Autodesk Fusion 360 part; units mm, degrees
(part 2 of 9)
sketch "草图7 (4)" plane through (0, 0, 36) normal (0, 0, 1) x (1, 0, 0) in component "L2_RemovableGrate"
  line L0 (299, 60.3) -> (303, 60.3)
  line L1 (303, 60.3) -> (303, 129.7)
  line L2 (303, 129.7) -> (299, 129.7)
  line L3 (299, 129.7) -> (299, 60.3)
  dimension "d526" = 299
  dimension "d528" = 4
  dimension "d529" = 69.4
  constraint horizontal L0
  constraint vertical L1
  constraint horizontal L2
  constraint vertical L3
  measures "d526" horizontal distance of origin L0.start
  measures "d528" horizontal distance of L0.start L0.end
  measures "d529" vertical distance of L0.end L1.end
extrude "Drain slot 6'" cut sketch "草图7 (4)" along normal blind 4 bodies 8 in component "L2_RemovableGrate"
ref_plane "工作平面8" through (0, 0, 36) normal (0, 0, 1) x (1, 0, 0) in component "L2_RemovableGrate"
sketch "草图8 (4)" plane through (0, 0, 36) normal (0, 0, 1) x (1, 0, 0) in component "L2_RemovableGrate"
  line L0 (309, 60.3) -> (313, 60.3)
  line L1 (313, 60.3) -> (313, 129.7)
  line L2 (313, 129.7) -> (309, 129.7)
  line L3 (309, 129.7) -> (309, 60.3)
  dimension "d534" = 309
  dimension "d536" = 4
  dimension "d537" = 69.4
  constraint horizontal L0
  constraint vertical L1
  constraint horizontal L2
  constraint vertical L3
  measures "d534" horizontal distance of origin L0.start
  measures "d536" horizontal distance of L0.start L0.end
  measures "d537" vertical distance of L0.end L1.end
extrude "Drain slot 7'" cut sketch "草图8 (4)" along normal blind 4 bodies 8 in component "L2_RemovableGrate"
ref_plane "工作平面9" through (0, 0, 36) normal (0, 0, 1) x (1, 0, 0) in component "L2_RemovableGrate"
sketch "草图9 (4)" plane through (0, 0, 36) normal (0, 0, 1) x (1, 0, 0) in component "L2_RemovableGrate"
  line L0 (319, 60.3) -> (323, 60.3)
  line L1 (323, 60.3) -> (323, 129.7)
  line L2 (323, 129.7) -> (319, 129.7)
  line L3 (319, 129.7) -> (319, 60.3)
  dimension "d542" = 319
  dimension "d544" = 4
  dimension "d545" = 69.4
  constraint horizontal L0
  constraint vertical L1
  constraint horizontal L2
  constraint vertical L3
  measures "d542" horizontal distance of origin L0.start
  measures "d544" horizontal distance of L0.start L0.end
  measures "d545" vertical distance of L0.end L1.end
extrude "Drain slot 8'" cut sketch "草图9 (4)" along normal blind 4 bodies 8 in component "L2_RemovableGrate"
ref_plane "工作平面10" through (0, 0, 36) normal (0, 0, 1) x (1, 0, 0) in component "L2_RemovableGrate"
sketch "草图10 (4)" plane through (0, 0, 36) normal (0, 0, 1) x (1, 0, 0) in component "L2_RemovableGrate"
  line L0 (329, 60.3) -> (333, 60.3)
  line L1 (333, 60.3) -> (333, 129.7)
  line L2 (333, 129.7) -> (329, 129.7)
  line L3 (329, 129.7) -> (329, 60.3)
  dimension "d550" = 329
  dimension "d552" = 4
  dimension "d553" = 69.4
  constraint horizontal L0
  constraint vertical L1
  constraint horizontal L2
  constraint vertical L3
  measures "d550" horizontal distance of origin L0.start
  measures "d552" horizontal distance of L0.start L0.end
  measures "d553" vertical distance of L0.end L1.end
extrude "Drain slot 9'" cut sketch "草图10 (4)" along normal blind 4 bodies 8 in component "L2_RemovableGrate"
ref_plane "工作平面11" through (0, 0, 36) normal (0, 0, 1) x (1, 0, 0) in component "L2_RemovableGrate"
sketch "草图11 (4)" plane through (0, 0, 36) normal (0, 0, 1) x (1, 0, 0) in component "L2_RemovableGrate"
  line L0 (339, 60.3) -> (343, 60.3)
  line L1 (343, 60.3) -> (343, 129.7)
  line L2 (343, 129.7) -> (339, 129.7)
  line L3 (339, 129.7) -> (339, 60.3)
  dimension "d558" = 339
  dimension "d560" = 4
  dimension "d561" = 69.4
  constraint horizontal L0
  constraint vertical L1
  constraint horizontal L2
  constraint vertical L3
  measures "d558" horizontal distance of origin L0.start
  measures "d560" horizontal distance of L0.start L0.end
  measures "d561" vertical distance of L0.end L1.end
extrude "Drain slot 10'" cut sketch "草图11 (4)" along normal blind 4 bodies 8 in component "L2_RemovableGrate"
ref_plane "工作平面12" through (0, 0, 36) normal (0, 0, 1) x (1, 0, 0) in component "L2_RemovableGrate"
sketch "草图12 (4)" plane through (0, 0, 36) normal (0, 0, 1) x (1, 0, 0) in component "L2_RemovableGrate"
  line L0 (349, 60.3) -> (353, 60.3)
  line L1 (353, 60.3) -> (353, 129.7)
  line L2 (353, 129.7) -> (349, 129.7)
  line L3 (349, 129.7) -> (349, 60.3)
  dimension "d566" = 349
  dimension "d568" = 4
  dimension "d569" = 69.4
  constraint horizontal L0
  constraint vertical L1
  constraint horizontal L2
  constraint vertical L3
  measures "d566" horizontal distance of origin L0.start
  measures "d568" horizontal distance of L0.start L0.end
  measures "d569" vertical distance of L0.end L1.end
extrude "Drain slot 11'" cut sketch "草图12 (4)" along normal blind 4 bodies 8 in component "L2_RemovableGrate"
ref_plane "工作平面13" through (0, 0, 36) normal (0, 0, 1) x (1, 0, 0) in component "L2_RemovableGrate"
sketch "草图13 (4)" plane through (0, 0, 36) normal (0, 0, 1) x (1, 0, 0) in component "L2_RemovableGrate"
  line L0 (359, 60.3) -> (363, 60.3)
  line L1 (363, 60.3) -> (363, 129.7)
  line L2 (363, 129.7) -> (359, 129.7)
  line L3 (359, 129.7) -> (359, 60.3)
  dimension "d574" = 359
  dimension "d576" = 4
  dimension "d577" = 69.4
  constraint horizontal L0
  constraint vertical L1
  constraint horizontal L2
  constraint vertical L3
  measures "d574" horizontal distance of origin L0.start
  measures "d576" horizontal distance of L0.start L0.end
  measures "d577" vertical distance of L0.end L1.end
extrude "Drain slot 12'" cut sketch "草图13 (4)" along normal blind 4 bodies 8 in component "L2_RemovableGrate"
ref_plane "工作平面14" through (0, 0, 36) normal (0, 0, 1) x (1, 0, 0) in component "L2_RemovableGrate"
sketch "草图14 (4)" plane through (0, 0, 36) normal (0, 0, 1) x (1, 0, 0) in component "L2_RemovableGrate"
  line L0 (369, 60.3) -> (373, 60.3)
  line L1 (373, 60.3) -> (373, 129.7)
  line L2 (373, 129.7) -> (369, 129.7)
  line L3 (369, 129.7) -> (369, 60.3)
  dimension "d582" = 369
  dimension "d584" = 4
  dimension "d585" = 69.4
  constraint horizontal L0
  constraint vertical L1
  constraint horizontal L2
  constraint vertical L3
  measures "d582" horizontal distance of origin L0.start
  measures "d584" horizontal distance of L0.start L0.end
  measures "d585" vertical distance of L0.end L1.end
extrude "Drain slot 13'" cut sketch "草图14 (4)" along normal blind 4 bodies 8 in component "L2_RemovableGrate"
ref_plane "工作平面15" through (0, 0, 36) normal (0, 0, 1) x (1, 0, 0) in component "L2_RemovableGrate"
sketch "草图15 (4)" plane through (0, 0, 36) normal (0, 0, 1) x (1, 0, 0) in component "L2_RemovableGrate"
  line L0 (379, 60.3) -> (383, 60.3)
  line L1 (383, 60.3) -> (383, 129.7)
  line L2 (383, 129.7) -> (379, 129.7)
  line L3 (379, 129.7) -> (379, 60.3)
  dimension "d590" = 379
  dimension "d592" = 4
  dimension "d593" = 69.4
  constraint horizontal L0
  constraint vertical L1
  constraint horizontal L2
  constraint vertical L3
  measures "d590" horizontal distance of origin L0.start
  measures "d592" horizontal distance of L0.start L0.end
  measures "d593" vertical distance of L0.end L1.end
extrude "Drain slot 14" cut sketch "草图15 (4)" along normal blind 4 bodies 8 in component "L2_RemovableGrate"
ref_plane "工作平面16" through (0, 0, 36) normal (0, 0, 1) x (1, 0, 0) in component "L2_RemovableGrate"
sketch "草图16" plane through (0, 0, 36) normal (0, 0, 1) x (1, 0, 0) in component "L2_RemovableGrate"
  line L0 (389, 60.3) -> (393, 60.3)
  line L1 (393, 60.3) -> (393, 129.7)
  line L2 (393, 129.7) -> (389, 129.7)
  line L3 (389, 129.7) -> (389, 60.3)
  dimension "d598" = 389
  dimension "d600" = 4
  dimension "d601" = 69.4
  constraint horizontal L0
  constraint vertical L1
  constraint horizontal L2
  constraint vertical L3
  measures "d598" horizontal distance of origin L0.start
  measures "d600" horizontal distance of L0.start L0.end
  measures "d601" vertical distance of L0.end L1.end
extrude "Drain slot 15" cut sketch "草图16" along normal blind 4 bodies 8 in component "L2_RemovableGrate"
ref_plane "工作平面17" through (0, 0, 36) normal (0, 0, 1) x (1, 0, 0) in component "L2_RemovableGrate"
sketch "草图17" plane through (0, 0, 36) normal (0, 0, 1) x (1, 0, 0) in component "L2_RemovableGrate"
  line L0 (399, 60.3) -> (403, 60.3)
  line L1 (403, 60.3) -> (403, 129.7)
  line L2 (403, 129.7) -> (399, 129.7)
  line L3 (399, 129.7) -> (399, 60.3)
  dimension "d606" = 399
  dimension "d608" = 4
  dimension "d609" = 69.4
  constraint horizontal L0
  constraint vertical L1
  constraint horizontal L2
  constraint vertical L3
  measures "d606" horizontal distance of origin L0.start
  measures "d608" horizontal distance of L0.start L0.end
  measures "d609" vertical distance of L0.end L1.end
extrude "Drain slot 16" cut sketch "草图17" along normal blind 4 bodies 8 in component "L2_RemovableGrate"
ref_plane "工作平面18" through (0, 0, 36) normal (0, 0, 1) x (1, 0, 0) in component "L2_RemovableGrate"
sketch "草图18" plane through (0, 0, 36) normal (0, 0, 1) x (1, 0, 0) in component "L2_RemovableGrate"
  line L0 (409, 60.3) -> (413, 60.3)
  line L1 (413, 60.3) -> (413, 129.7)
  line L2 (413, 129.7) -> (409, 129.7)
  line L3 (409, 129.7) -> (409, 60.3)
  dimension "d614" = 409
  dimension "d616" = 4
  dimension "d617" = 69.4
  constraint horizontal L0
  constraint vertical L1
  constraint horizontal L2
  constraint vertical L3
  measures "d614" horizontal distance of origin L0.start
  measures "d616" horizontal distance of L0.start L0.end
  measures "d617" vertical distance of L0.end L1.end
extrude "Drain slot 17" cut sketch "草图18" along normal blind 4 bodies 8 in component "L2_RemovableGrate"
ref_plane "工作平面19" through (0, 0, 36) normal (0, 0, 1) x (1, 0, 0) in component "L2_RemovableGrate"
sketch "草图19" plane through (0, 0, 36) normal (0, 0, 1) x (1, 0, 0) in component "L2_RemovableGrate"
  line L0 (323, 132.7) -> (339, 132.7)
  line L1 (339, 132.7) -> (339, 137.7)
  line L2 (339, 137.7) -> (323, 137.7)
  line L3 (323, 137.7) -> (323, 132.7)
  dimension "d622" = 323
  dimension "d623" = 132.7
  dimension "d624" = 16
  dimension "d625" = 5
  constraint horizontal L0
  constraint vertical L1
  constraint horizontal L2
  constraint vertical L3
  measures "d622" horizontal distance of origin L0.start
  measures "d623" vertical distance of origin L0.start
  measures "d624" horizontal distance of L0.start L0.end
  measures "d625" vertical distance of L0.end L1.end
extrude "Finger lift notch'" cut sketch "草图19" along normal blind 4 bodies 8 in component "L2_RemovableGrate"
ref_plane "工作平面1" through (0, 0, 0) normal (0, 0, 1) x (1, 0, 0) in component "L2_Foot_00"
sketch "草图1 (9)" plane through (0, 0, 0) normal (0, 0, 1) x (1, 0, 0) in component "L2_Foot_00"
  line L0 (235, 53) -> (251, 53)
  line L1 (251, 53) -> (251, 69)
  line L2 (251, 69) -> (235, 69)
  line L3 (235, 69) -> (235, 53)
  dimension "d630" = 235
  dimension "d631" = 53
  dimension "d632" = 16
  dimension "d633" = 16
  constraint horizontal L0
  constraint vertical L1
  constraint horizontal L2
  constraint vertical L3
  measures "d630" horizontal distance of origin L0.start
  measures "d631" vertical distance of origin L0.start
  measures "d632" horizontal distance of L0.start L0.end
  measures "d633" vertical distance of L0.end L1.end
extrude "Foot base''''" add sketch "草图1 (9)" along normal blind 20 separate body makes body 9 in component "L2_Foot_00"
ref_plane "工作平面2" through (0, 0, 20) normal (0, 0, 1) x (1, 0, 0) in component "L2_Foot_00"
sketch "草图2 (9)" plane through (0, 0, 20) normal (0, 0, 1) x (1, 0, 0) in component "L2_Foot_00"
  line L0 (239, 57) -> (247, 57)
  line L1 (247, 57) -> (247, 65)
  line L2 (247, 65) -> (239, 65)
  line L3 (239, 65) -> (239, 57)
  dimension "d638" = 239
  dimension "d639" = 57
  dimension "d640" = 8
  dimension "d641" = 8
  constraint horizontal L0
  constraint vertical L1
  constraint horizontal L2
  constraint vertical L3
  measures "d638" horizontal distance of origin L0.start
  measures "d639" vertical distance of origin L0.start
  measures "d640" horizontal distance of L0.start L0.end
  measures "d641" vertical distance of L0.end L1.end
extrude "Locating peg''''" add sketch "草图2 (9)" along normal blind 1.5 bodies 9 in component "L2_Foot_00"
ref_plane "工作平面1" through (0, 0, 0) normal (0, 0, 1) x (1, 0, 0) in component "L2_Foot_01"
sketch "草图1 (10)" plane through (0, 0, 0) normal (0, 0, 1) x (1, 0, 0) in component "L2_Foot_01"
  line L0 (235, 115) -> (251, 115)
  line L1 (251, 115) -> (251, 131)
  line L2 (251, 131) -> (235, 131)
  line L3 (235, 131) -> (235, 115)
  dimension "d646" = 235
  dimension "d647" = 115
  dimension "d648" = 16
  dimension "d649" = 16
  constraint horizontal L0
  constraint vertical L1
  constraint horizontal L2
  constraint vertical L3
  measures "d646" horizontal distance of origin L0.start
  measures "d647" vertical distance of origin L0.start
  measures "d648" horizontal distance of L0.start L0.end
  measures "d649" vertical distance of L0.end L1.end
extrude "Foot base'''''" add sketch "草图1 (10)" along normal blind 20 separate body makes body 10 in component "L2_Foot_01"
ref_plane "工作平面2" through (0, 0, 20) normal (0, 0, 1) x (1, 0, 0) in component "L2_Foot_01"
sketch "草图2 (10)" plane through (0, 0, 20) normal (0, 0, 1) x (1, 0, 0) in component "L2_Foot_01"
  line L0 (239, 119) -> (247, 119)
  line L1 (247, 119) -> (247, 127)
  line L2 (247, 127) -> (239, 127)
  line L3 (239, 127) -> (239, 119)
  dimension "d654" = 239
  dimension "d655" = 119
  dimension "d656" = 8
  dimension "d657" = 8
  constraint horizontal L0
  constraint vertical L1
  constraint horizontal L2
  constraint vertical L3
  measures "d654" horizontal distance of origin L0.start
  measures "d655" vertical distance of origin L0.start
  measures "d656" horizontal distance of L0.start L0.end
  measures "d657" vertical distance of L0.end L1.end
extrude "Locating peg'''''" add sketch "草图2 (10)" along normal blind 1.5 bodies 10 in component "L2_Foot_01"
ref_plane "工作平面1" through (0, 0, 0) normal (0, 0, 1) x (1, 0, 0) in component "L2_Foot_10"
sketch "草图1 (11)" plane through (0, 0, 0) normal (0, 0, 1) x (1, 0, 0) in component "L2_Foot_10"
  line L0 (411, 53) -> (427, 53)
  line L1 (427, 53) -> (427, 69)
  line L2 (427, 69) -> (411, 69)
  line L3 (411, 69) -> (411, 53)
  dimension "d662" = 411
  dimension "d663" = 53
  dimension "d664" = 16
  dimension "d665" = 16
  constraint horizontal L0
  constraint vertical L1
  constraint horizontal L2
  constraint vertical L3
  measures "d662" horizontal distance of origin L0.start
  measures "d663" vertical distance of origin L0.start
  measures "d664" horizontal distance of L0.start L0.end
  measures "d665" vertical distance of L0.end L1.end
extrude "Foot base''''''" add sketch "草图1 (11)" along normal blind 20 separate body makes body 11 in component "L2_Foot_10"
ref_plane "工作平面2" through (0, 0, 20) normal (0, 0, 1) x (1, 0, 0) in component "L2_Foot_10"
sketch "草图2 (11)" plane through (0, 0, 20) normal (0, 0, 1) x (1, 0, 0) in component "L2_Foot_10"
  line L0 (415, 57) -> (423, 57)
  line L1 (423, 57) -> (423, 65)
  line L2 (423, 65) -> (415, 65)
  line L3 (415, 65) -> (415, 57)
  dimension "d670" = 415
  dimension "d671" = 57
  dimension "d672" = 8
  dimension "d673" = 8
  constraint horizontal L0
  constraint vertical L1
  constraint horizontal L2
  constraint vertical L3
  measures "d670" horizontal distance of origin L0.start
  measures "d671" vertical distance of origin L0.start
  measures "d672" horizontal distance of L0.start L0.end
  measures "d673" vertical distance of L0.end L1.end
extrude "Locating peg''''''" add sketch "草图2 (11)" along normal blind 1.5 bodies 11 in component "L2_Foot_10"
ref_plane "工作平面1" through (0, 0, 0) normal (0, 0, 1) x (1, 0, 0) in component "L2_Foot_11"
sketch "草图1 (12)" plane through (0, 0, 0) normal (0, 0, 1) x (1, 0, 0) in component "L2_Foot_11"
  line L0 (411, 115) -> (427, 115)
  line L1 (427, 115) -> (427, 131)
  line L2 (427, 131) -> (411, 131)
  line L3 (411, 131) -> (411, 115)
  dimension "d678" = 411
  dimension "d679" = 115
  dimension "d680" = 16
  dimension "d681" = 16
  constraint horizontal L0
  constraint vertical L1
  constraint horizontal L2
  constraint vertical L3
  measures "d678" horizontal distance of origin L0.start
  measures "d679" vertical distance of origin L0.start
  measures "d680" horizontal distance of L0.start L0.end
  measures "d681" vertical distance of L0.end L1.end
extrude "Foot base'''''''" add sketch "草图1 (12)" along normal blind 20 separate body makes body 12 in component "L2_Foot_11"
ref_plane "工作平面2" through (0, 0, 20) normal (0, 0, 1) x (1, 0, 0) in component "L2_Foot_11"
sketch "草图2 (12)" plane through (0, 0, 20) normal (0, 0, 1) x (1, 0, 0) in component "L2_Foot_11"
  line L0 (415, 119) -> (423, 119)
  line L1 (423, 119) -> (423, 127)
  line L2 (423, 127) -> (415, 127)
  line L3 (415, 127) -> (415, 119)
  dimension "d686" = 415
  dimension "d687" = 119
  dimension "d688" = 8
  dimension "d689" = 8
  constraint horizontal L0
  constraint vertical L1
  constraint horizontal L2
  constraint vertical L3
  measures "d686" horizontal distance of origin L0.start
  measures "d687" vertical distance of origin L0.start
  measures "d688" horizontal distance of L0.start L0.end
  measures "d689" vertical distance of L0.end L1.end
extrude "Locating peg'''''''" add sketch "草图2 (12)" along normal blind 1.5 bodies 12 in component "L2_Foot_11"
ref_plane "工作平面1" through (0, 0, 20) normal (0, 0, 1) x (1, 0, 0) in component "R1_DrainPan"
sketch "草图1 (13)" plane through (0, 0, 20) normal (0, 0, 1) x (1, 0, 0) in component "R1_DrainPan"
  line L0 (590, 50) -> (724, 50)
  line L1 (724, 50) -> (724, 140)
  line L2 (724, 140) -> (590, 140)
  line L3 (590, 140) -> (590, 50)
  dimension "d694" = 590
  dimension "d695" = 50
  dimension "d696" = 134
  dimension "d697" = 90
  constraint horizontal L0
  constraint vertical L1
  constraint horizontal L2
  constraint vertical L3
  measures "d694" horizontal distance of origin L0.start
  measures "d695" vertical distance of origin L0.start
  measures "d696" horizontal distance of L0.start L0.end
  measures "d697" vertical distance of L0.end L1.end
extrude "Pan blank''" add sketch "草图1 (13)" along normal blind 20 separate body makes body 13 in component "R1_DrainPan"
fillet "Outside corner rounds''" radius 3 4 edges at (590, 140, 30) (724, 140, 30) (724, 50, 30) (590, 50, 30) on bodies 13 in component "R1_DrainPan"
ref_plane "工作平面2" through (593, 0, 0) normal (1, 0, 0) x (0, 1, 0) in component "R1_DrainPan"
sketch "草图2 (13)" plane through (593, 0, 0) normal (1, 0, 0) x (0, 0, -1) in component "R1_DrainPan"
  line L0 (-30.8318, 53) -> (-24.958, 137)
  line L1 (-24.958, 137) -> (-41, 137)
  line L2 (-41, 137) -> (-41, 53)
  line L3 (-41, 53) -> (-30.8318, 53)
  dimension "d704" = 30.8318
  dimension "d706" = 24.958
  dimension "d708" = 41
  constraint horizontal L1
  constraint vertical L2
  constraint horizontal L3
  measures "d704" horizontal distance of origin L0.start
  measures "d706" horizontal distance of origin L0.end
  measures "d708" horizontal distance of origin L1.end
extrude "Sloped catch cavity''" cut sketch "草图2 (13)" along normal blind 128 bodies 13 in component "R1_DrainPan"
ref_plane "工作平面3" through (640, 0, 0) normal (1, 0, 0) x (0, 1, 0) in component "R1_DrainPan"
sketch "草图3 (5)" plane through (640, 0, 0) normal (1, 0, 0) x (0, 0, -1) in component "R1_DrainPan"
  line L0 (-20, 137) -> (-20, 165)
  line L1 (-20, 165) -> (-23, 165)
  line L2 (-23, 165) -> (-24.958, 137)
  line L3 (-24.958, 137) -> (-20, 137)
  dimension "d716" = 23
  dimension "d717" = 24.958
  constraint vertical L0
  constraint horizontal L1
  constraint horizontal L3
  measures "d716" horizontal distance of origin L1.end
  measures "d717" horizontal distance of origin L2.end
extrude "Drain tongue floor''" add sketch "草图3 (5)" along normal blind 34 bodies 13 in component "R1_DrainPan"
ref_plane "工作平面4" through (640, 0, 0) normal (1, 0, 0) x (0, 1, 0) in component "R1_DrainPan"
sketch "草图4 (5)" plane through (640, 0, 0) normal (1, 0, 0) x (0, 0, -1) in component "R1_DrainPan"
  line L0 (-20, 137) -> (-20, 165)
  line L1 (-20, 165) -> (-29, 165)
  line L2 (-29, 165) -> (-30.958, 137)
  line L3 (-30.958, 137) -> (-20, 137)
  dimension "d725" = 29
  dimension "d726" = 30.958
  constraint vertical L0
  constraint horizontal L1
  constraint horizontal L3
  measures "d725" horizontal distance of origin L1.end
  measures "d726" horizontal distance of origin L2.end
extrude "Tongue side rail''" add sketch "草图4 (5)" along normal blind 3 bodies 13 in component "R1_DrainPan"
ref_plane "工作平面5" through (671, 0, 0) normal (1, 0, 0) x (0, 1, 0) in component "R1_DrainPan"
sketch "草图5 (5)" plane through (671, 0, 0) normal (1, 0, 0) x (0, 0, -1) in component "R1_DrainPan"
  line L0 (-20, 137) -> (-20, 165)
  line L1 (-20, 165) -> (-29, 165)
  line L2 (-29, 165) -> (-30.958, 137)
  line L3 (-30.958, 137) -> (-20, 137)
  dimension "d734" = 29
  dimension "d735" = 30.958
  constraint vertical L0
  constraint horizontal L1
  constraint horizontal L3
  measures "d734" horizontal distance of origin L1.end
  measures "d735" horizontal distance of origin L2.end
extrude "Tongue side rail (1)''" add sketch "草图5 (5)" along normal blind 3 bodies 13 in component "R1_DrainPan"
ref_plane "工作平面6" through (643, 0, 0) normal (1, 0, 0) x (0, 1, 0) in component "R1_DrainPan"
sketch "草图6 (5)" plane through (643, 0, 0) normal (1, 0, 0) x (0, 0, -1) in component "R1_DrainPan"
  line L0 (-24.958, 137) -> (-23, 165)
  line L1 (-23, 165) -> (-41, 165)
  line L2 (-41, 165) -> (-41, 137)
  line L3 (-41, 137) -> (-24.958, 137)
  dimension "d740" = 24.958
  dimension "d742" = 23
  dimension "d744" = 41
  constraint horizontal L1
  constraint vertical L2
  constraint horizontal L3
  measures "d740" horizontal distance of origin L0.start
  measures "d742" horizontal distance of origin L0.end
  measures "d744" horizontal distance of origin L1.end
extrude "Open drain mouth''" cut sketch "草图6 (5)" along normal blind 28 bodies 13 in component "R1_DrainPan"
ref_plane "工作平面7" through (0, 0, 20) normal (0, 0, 1) x (1, 0, 0) in component "R1_DrainPan"
sketch "草图7 (5)" plane through (0, 0, 20) normal (0, 0, 1) x (1, 0, 0) in component "R1_DrainPan"
  line L0 (593, 53) -> (605, 53)
  line L1 (605, 53) -> (605, 65)
  line L2 (605, 65) -> (593, 65)
  line L3 (593, 65) -> (593, 53)
  dimension "d751" = 12
  dimension "d752" = 12
  constraint horizontal L0
  constraint vertical L1
  constraint horizontal L2
  constraint vertical L3
  measures "d751" horizontal distance of L0.start L0.end
  measures "d752" vertical distance of L0.end L1.end
extrude "Grate seat 00''" add sketch "草图7 (5)" along normal blind 16 bodies 13 in component "R1_DrainPan"
ref_plane "工作平面8" through (0, 0, 20) normal (0, 0, 1) x (1, 0, 0) in component "R1_DrainPan"
sketch "草图8 (5)" plane through (0, 0, 20) normal (0, 0, 1) x (1, 0, 0) in component "R1_DrainPan"
  line L0 (593, 125) -> (605, 125)
  line L1 (605, 125) -> (605, 137)
  line L2 (605, 137) -> (593, 137)
  line L3 (593, 137) -> (593, 125)
  dimension "d758" = 125
  dimension "d759" = 12
  dimension "d760" = 12
  constraint horizontal L0
  constraint vertical L1
  constraint horizontal L2
  constraint vertical L3
  measures "d758" vertical distance of origin L0.start
  measures "d759" horizontal distance of L0.start L0.end
  measures "d760" vertical distance of L0.end L1.end
extrude "Grate seat 01''" add sketch "草图8 (5)" along normal blind 16 bodies 13 in component "R1_DrainPan"
ref_plane "工作平面9" through (0, 0, 20) normal (0, 0, 1) x (1, 0, 0) in component "R1_DrainPan"
sketch "草图9 (5)" plane through (0, 0, 20) normal (0, 0, 1) x (1, 0, 0) in component "R1_DrainPan"
  line L0 (709, 53) -> (721, 53)
  line L1 (721, 53) -> (721, 65)
  line L2 (721, 65) -> (709, 65)
  line L3 (709, 65) -> (709, 53)
  dimension "d765" = 709
  dimension "d767" = 12
  dimension "d768" = 12
  constraint horizontal L0
  constraint vertical L1
  constraint horizontal L2
  constraint vertical L3
  measures "d765" horizontal distance of origin L0.start
  measures "d767" horizontal distance of L0.start L0.end
  measures "d768" vertical distance of L0.end L1.end
extrude "Grate seat 10''" add sketch "草图9 (5)" along normal blind 16 bodies 13 in component "R1_DrainPan"
ref_plane "工作平面10" through (0, 0, 20) normal (0, 0, 1) x (1, 0, 0) in component "R1_DrainPan"
sketch "草图10 (5)" plane through (0, 0, 20) normal (0, 0, 1) x (1, 0, 0) in component "R1_DrainPan"
  line L0 (709, 125) -> (721, 125)
  line L1 (721, 125) -> (721, 137)
  line L2 (721, 137) -> (709, 137)
  line L3 (709, 137) -> (709, 125)
  dimension "d773" = 709
  dimension "d774" = 125
  dimension "d775" = 12
  dimension "d776" = 12
  constraint horizontal L0
  constraint vertical L1
  constraint horizontal L2
  constraint vertical L3
  measures "d773" horizontal distance of origin L0.start
  measures "d774" vertical distance of origin L0.start
  measures "d775" horizontal distance of L0.start L0.end
  measures "d776" vertical distance of L0.end L1.end
extrude "Grate seat 11''" add sketch "草图10 (5)" along normal blind 16 bodies 13 in component "R1_DrainPan"
ref_plane "工作平面11" through (640, 0, 0) normal (1, 0, 0) x (0, 1, 0) in component "R1_DrainPan"
sketch "草图11 (5)" plane through (640, 0, 0) normal (1, 0, 0) x (0, 0, -1) in component "R1_DrainPan"
  line L0 (-19.8, 163) -> (-19.8, 164)
  line L1 (-19.8, 164) -> (-20.6, 164)
  line L2 (-20.6, 164) -> (-20.6, 163)
  line L3 (-20.6, 163) -> (-19.8, 163)
  dimension "d781" = 19.8
  dimension "d782" = 163
  dimension "d783" = 164
  dimension "d784" = 20.6
  constraint vertical L0
  constraint horizontal L1
  constraint vertical L2
  constraint horizontal L3
  measures "d781" horizontal distance of origin L0.start
  measures "d782" vertical distance of origin L0.start
  measures "d783" vertical distance of origin L0.end
  measures "d784" horizontal distance of origin L1.end
extrude "Drip break underside groove''" cut sketch "草图11 (5)" along normal blind 34 bodies 13 in component "R1_DrainPan"
ref_plane "工作平面12" through (0, 0, 20) normal (0, 0, 1) x (1, 0, 0) in component "R1_DrainPan"
sketch "草图12 (5)" plane through (0, 0, 20) normal (0, 0, 1) x (1, 0, 0) in component "R1_DrainPan"
  line L0 (596.75, 56.75) -> (605.25, 56.75)
  line L1 (605.25, 56.75) -> (605.25, 65.25)
  line L2 (605.25, 65.25) -> (596.75, 65.25)
  line L3 (596.75, 65.25) -> (596.75, 56.75)
  dimension "d789" = 596.75
  dimension "d790" = 56.75
  dimension "d791" = 8.5
  dimension "d792" = 8.5
  constraint horizontal L0
  constraint vertical L1
  constraint horizontal L2
  constraint vertical L3
  measures "d789" horizontal distance of origin L0.start
  measures "d790" vertical distance of origin L0.start
  measures "d791" horizontal distance of L0.start L0.end
  measures "d792" vertical distance of L0.end L1.end
extrude "Foot socket 00''" cut sketch "草图12 (5)" along normal blind 1.8 bodies 13 in component "R1_DrainPan"
ref_plane "工作平面13" through (0, 0, 20) normal (0, 0, 1) x (1, 0, 0) in component "R1_DrainPan"
sketch "草图13 (5)" plane through (0, 0, 20) normal (0, 0, 1) x (1, 0, 0) in component "R1_DrainPan"
  line L0 (596.75, 118.75) -> (605.25, 118.75)
  line L1 (605.25, 118.75) -> (605.25, 127.25)
  line L2 (605.25, 127.25) -> (596.75, 127.25)
  line L3 (596.75, 127.25) -> (596.75, 118.75)
  dimension "d797" = 596.75
  dimension "d798" = 118.75
  dimension "d799" = 8.5
  dimension "d800" = 8.5
  constraint horizontal L0
  constraint vertical L1
  constraint horizontal L2
  constraint vertical L3
  measures "d797" horizontal distance of origin L0.start
  measures "d798" vertical distance of origin L0.start
  measures "d799" horizontal distance of L0.start L0.end
  measures "d800" vertical distance of L0.end L1.end
extrude "Foot socket 01''" cut sketch "草图13 (5)" along normal blind 1.8 bodies 13 in component "R1_DrainPan"
ref_plane "工作平面14" through (0, 0, 20) normal (0, 0, 1) x (1, 0, 0) in component "R1_DrainPan"
sketch "草图14 (5)" plane through (0, 0, 20) normal (0, 0, 1) x (1, 0, 0) in component "R1_DrainPan"
  line L0 (708.75, 56.75) -> (717.25, 56.75)
  line L1 (717.25, 56.75) -> (717.25, 65.25)
  line L2 (717.25, 65.25) -> (708.75, 65.25)
  line L3 (708.75, 65.25) -> (708.75, 56.75)
  dimension "d805" = 708.75
  dimension "d806" = 56.75
  dimension "d807" = 8.5
  dimension "d808" = 8.5
  constraint horizontal L0
  constraint vertical L1
  constraint horizontal L2
  constraint vertical L3
  measures "d805" horizontal distance of origin L0.start
  measures "d806" vertical distance of origin L0.start
  measures "d807" horizontal distance of L0.start L0.end
  measures "d808" vertical distance of L0.end L1.end
extrude "Foot socket 10''" cut sketch "草图14 (5)" along normal blind 1.8 bodies 13 in component "R1_DrainPan"
ref_plane "工作平面15" through (0, 0, 20) normal (0, 0, 1) x (1, 0, 0) in component "R1_DrainPan"
sketch "草图15 (5)" plane through (0, 0, 20) normal (0, 0, 1) x (1, 0, 0) in component "R1_DrainPan"
  line L0 (708.75, 118.75) -> (717.25, 118.75)
  line L1 (717.25, 118.75) -> (717.25, 127.25)
  line L2 (717.25, 127.25) -> (708.75, 127.25)
  line L3 (708.75, 127.25) -> (708.75, 118.75)
  dimension "d813" = 708.75
  dimension "d814" = 118.75
  dimension "d815" = 8.5
  dimension "d816" = 8.5
  constraint horizontal L0
  constraint vertical L1
  constraint horizontal L2
  constraint vertical L3
  measures "d813" horizontal distance of origin L0.start
  measures "d814" vertical distance of origin L0.start
  measures "d815" horizontal distance of L0.start L0.end
  measures "d764" distance of L0.end L1.end
extrude "Foot socket 11''" cut sketch "草图15 (5)" along normal blind 1.8 bodies 13 in component "R1_DrainPan"
ref_plane "工作平面1" through (0, 0, 36) normal (0, 0, 1) x (1, 0, 0) in component "R1_RemovableGrate"
sketch "草图1 (14)" plane through (0, 0, 36) normal (0, 0, 1) x (1, 0, 0) in component "R1_RemovableGrate"
  line L0 (593.3, 53.3) -> (720.7, 53.3)
  line L1 (720.7, 53.3) -> (720.7, 136.7)
  line L2 (720.7, 136.7) -> (593.3, 136.7)
  line L3 (593.3, 136.7) -> (593.3, 53.3)
  dimension "d823" = 127.4
  dimension "d824" = 83.4
  constraint horizontal L0
  constraint vertical L1
  constraint horizontal L2
  constraint vertical L3
  measures "d823" horizontal distance of L0.start L0.end
  measures "d824" vertical distance of L0.end L1.end
extrude "Horizontal removable deck''" add sketch "草图1 (14)" along normal blind 4 separate body makes body 14 in component "R1_RemovableGrate"
ref_plane "工作平面2" through (0, 0, 36) normal (0, 0, 1) x (1, 0, 0) in component "R1_RemovableGrate"
sketch "草图2 (14)" plane through (0, 0, 36) normal (0, 0, 1) x (1, 0, 0) in component "R1_RemovableGrate"
  line L0 (605, 60.3) -> (609, 60.3)
  line L1 (609, 60.3) -> (609, 129.7)
  line L2 (609, 129.7) -> (605, 129.7)
  line L3 (605, 129.7) -> (605, 60.3)
  dimension "d829" = 605
  dimension "d831" = 4
  dimension "d832" = 69.4
  constraint horizontal L0
  constraint vertical L1
  constraint horizontal L2
  constraint vertical L3
  measures "d829" horizontal distance of origin L0.start
  measures "d831" horizontal distance of L0.start L0.end
  measures "d832" vertical distance of L0.end L1.end
extrude "Drain slot 1''" cut sketch "草图2 (14)" along normal blind 4 bodies 14 in component "R1_RemovableGrate"
ref_plane "工作平面3" through (0, 0, 36) normal (0, 0, 1) x (1, 0, 0) in component "R1_RemovableGrate"
sketch "草图3 (6)" plane through (0, 0, 36) normal (0, 0, 1) x (1, 0, 0) in component "R1_RemovableGrate"
  line L0 (615, 60.3) -> (619, 60.3)
  line L1 (619, 60.3) -> (619, 129.7)
  line L2 (619, 129.7) -> (615, 129.7)
  line L3 (615, 129.7) -> (615, 60.3)
  dimension "d837" = 615
  dimension "d839" = 4
  dimension "d840" = 69.4
  constraint horizontal L0
  constraint vertical L1
  constraint horizontal L2
  constraint vertical L3
  measures "d837" horizontal distance of origin L0.start
  measures "d839" horizontal distance of L0.start L0.end
  measures "d840" vertical distance of L0.end L1.end
extrude "Drain slot 2''" cut sketch "草图3 (6)" along normal blind 4 bodies 14 in component "R1_RemovableGrate"
ref_plane "工作平面4" through (0, 0, 36) normal (0, 0, 1) x (1, 0, 0) in component "R1_RemovableGrate"
sketch "草图4 (6)" plane through (0, 0, 36) normal (0, 0, 1) x (1, 0, 0) in component "R1_RemovableGrate"
  line L0 (625, 60.3) -> (629, 60.3)
  line L1 (629, 60.3) -> (629, 129.7)
  line L2 (629, 129.7) -> (625, 129.7)
  line L3 (625, 129.7) -> (625, 60.3)
  dimension "d845" = 625
  dimension "d847" = 4
  dimension "d848" = 69.4
  constraint horizontal L0
  constraint vertical L1
  constraint horizontal L2
  constraint vertical L3
  measures "d845" horizontal distance of origin L0.start
  measures "d847" horizontal distance of L0.start L0.end
  measures "d848" vertical distance of L0.end L1.end
extrude "Drain slot 3''" cut sketch "草图4 (6)" along normal blind 4 bodies 14 in component "R1_RemovableGrate"
ref_plane "工作平面5" through (0, 0, 36) normal (0, 0, 1) x (1, 0, 0) in component "R1_RemovableGrate"
sketch "草图5 (6)" plane through (0, 0, 36) normal (0, 0, 1) x (1, 0, 0) in component "R1_RemovableGrate"
  line L0 (635, 60.3) -> (639, 60.3)
  line L1 (639, 60.3) -> (639, 129.7)
  line L2 (639, 129.7) -> (635, 129.7)
  line L3 (635, 129.7) -> (635, 60.3)
  dimension "d853" = 635
  dimension "d855" = 4
  dimension "d856" = 69.4
  constraint horizontal L0
  constraint vertical L1
  constraint horizontal L2
  constraint vertical L3
  measures "d853" horizontal distance of origin L0.start
  measures "d855" horizontal distance of L0.start L0.end
  measures "d856" vertical distance of L0.end L1.end
extrude "Drain slot 4''" cut sketch "草图5 (6)" along normal blind 4 bodies 14 in component "R1_RemovableGrate"
ref_plane "工作平面6" through (0, 0, 36) normal (0, 0, 1) x (1, 0, 0) in component "R1_RemovableGrate"
sketch "草图6 (6)" plane through (0, 0, 36) normal (0, 0, 1) x (1, 0, 0) in component "R1_RemovableGrate"
  line L0 (645, 60.3) -> (649, 60.3)
  line L1 (649, 60.3) -> (649, 129.7)
  line L2 (649, 129.7) -> (645, 129.7)
  line L3 (645, 129.7) -> (645, 60.3)
  dimension "d861" = 645
  dimension "d863" = 4
  dimension "d864" = 69.4
  constraint horizontal L0
  constraint vertical L1
  constraint horizontal L2
  constraint vertical L3
  measures "d861" horizontal distance of origin L0.start
  measures "d863" horizontal distance of L0.start L0.end
  measures "d864" vertical distance of L0.end L1.end
extrude "Drain slot 5''" cut sketch "草图6 (6)" along normal blind 4 bodies 14 in component "R1_RemovableGrate"
ref_plane "工作平面7" through (0, 0, 36) normal (0, 0, 1) x (1, 0, 0) in component "R1_RemovableGrate"
sketch "草图7 (6)" plane through (0, 0, 36) normal (0, 0, 1) x (1, 0, 0) in component "R1_RemovableGrate"
  line L0 (655, 60.3) -> (659, 60.3)
  line L1 (659, 60.3) -> (659, 129.7)
  line L2 (659, 129.7) -> (655, 129.7)
  line L3 (655, 129.7) -> (655, 60.3)
  dimension "d869" = 655
  dimension "d871" = 4
  dimension "d872" = 69.4
  constraint horizontal L0
  constraint vertical L1
  constraint horizontal L2
  constraint vertical L3
  measures "d869" horizontal distance of origin L0.start
  measures "d871" horizontal distance of L0.start L0.end
  measures "d872" vertical distance of L0.end L1.end
extrude "Drain slot 6''" cut sketch "草图7 (6)" along normal blind 4 bodies 14 in component "R1_RemovableGrate"
ref_plane "工作平面8" through (0, 0, 36) normal (0, 0, 1) x (1, 0, 0) in component "R1_RemovableGrate"
sketch "草图8 (6)" plane through (0, 0, 36) normal (0, 0, 1) x (1, 0, 0) in component "R1_RemovableGrate"
  line L0 (665, 60.3) -> (669, 60.3)
  line L1 (669, 60.3) -> (669, 129.7)
  line L2 (669, 129.7) -> (665, 129.7)
  line L3 (665, 129.7) -> (665, 60.3)
  dimension "d877" = 665
  dimension "d879" = 4
  dimension "d880" = 69.4
  constraint horizontal L0
  constraint vertical L1
  constraint horizontal L2
  constraint vertical L3
  measures "d877" horizontal distance of origin L0.start
  measures "d879" horizontal distance of L0.start L0.end
  measures "d880" vertical distance of L0.end L1.end
extrude "Drain slot 7''" cut sketch "草图8 (6)" along normal blind 4 bodies 14 in component "R1_RemovableGrate"
ref_plane "工作平面9" through (0, 0, 36) normal (0, 0, 1) x (1, 0, 0) in component "R1_RemovableGrate"
sketch "草图9 (6)" plane through (0, 0, 36) normal (0, 0, 1) x (1, 0, 0) in component "R1_RemovableGrate"
  line L0 (675, 60.3) -> (679, 60.3)
  line L1 (679, 60.3) -> (679, 129.7)
  line L2 (679, 129.7) -> (675, 129.7)
  line L3 (675, 129.7) -> (675, 60.3)
  dimension "d885" = 675
  dimension "d887" = 4
  dimension "d888" = 69.4
  constraint horizontal L0
  constraint vertical L1
  constraint horizontal L2
  constraint vertical L3
  measures "d885" horizontal distance of origin L0.start
  measures "d887" horizontal distance of L0.start L0.end
  measures "d888" vertical distance of L0.end L1.end
extrude "Drain slot 8''" cut sketch "草图9 (6)" along normal blind 4 bodies 14 in component "R1_RemovableGrate"
ref_plane "工作平面10" through (0, 0, 36) normal (0, 0, 1) x (1, 0, 0) in component "R1_RemovableGrate"
sketch "草图10 (6)" plane through (0, 0, 36) normal (0, 0, 1) x (1, 0, 0) in component "R1_RemovableGrate"
  line L0 (685, 60.3) -> (689, 60.3)
  line L1 (689, 60.3) -> (689, 129.7)
  line L2 (689, 129.7) -> (685, 129.7)
  line L3 (685, 129.7) -> (685, 60.3)
  dimension "d893" = 685
  dimension "d895" = 4
  dimension "d896" = 69.4
  constraint horizontal L0
  constraint vertical L1
  constraint horizontal L2
  constraint vertical L3
  measures "d893" horizontal distance of origin L0.start
  measures "d895" horizontal distance of L0.start L0.end
  measures "d896" vertical distance of L0.end L1.end
extrude "Drain slot 9''" cut sketch "草图10 (6)" along normal blind 4 bodies 14 in component "R1_RemovableGrate"
ref_plane "工作平面11" through (0, 0, 36) normal (0, 0, 1) x (1, 0, 0) in component "R1_RemovableGrate"
sketch "草图11 (6)" plane through (0, 0, 36) normal (0, 0, 1) x (1, 0, 0) in component "R1_RemovableGrate"
  line L0 (695, 60.3) -> (699, 60.3)
  line L1 (699, 60.3) -> (699, 129.7)
  line L2 (699, 129.7) -> (695, 129.7)
  line L3 (695, 129.7) -> (695, 60.3)
  dimension "d901" = 695
  dimension "d903" = 4
  dimension "d904" = 69.4
  constraint horizontal L0
  constraint vertical L1
  constraint horizontal L2
  constraint vertical L3
  measures "d901" horizontal distance of origin L0.start
  measures "d903" horizontal distance of L0.start L0.end
  measures "d904" vertical distance of L0.end L1.end
extrude "Drain slot 10''" cut sketch "草图11 (6)" along normal blind 4 bodies 14 in component "R1_RemovableGrate"
ref_plane "工作平面12" through (0, 0, 36) normal (0, 0, 1) x (1, 0, 0) in component "R1_RemovableGrate"
sketch "草图12 (6)" plane through (0, 0, 36) normal (0, 0, 1) x (1, 0, 0) in component "R1_RemovableGrate"
  line L0 (705, 60.3) -> (709, 60.3)
  line L1 (709, 60.3) -> (709, 129.7)
  line L2 (709, 129.7) -> (705, 129.7)
  line L3 (705, 129.7) -> (705, 60.3)
  dimension "d909" = 705
  dimension "d911" = 4
  dimension "d912" = 69.4
  constraint horizontal L0
  constraint vertical L1
  constraint horizontal L2
  constraint vertical L3
  measures "d909" horizontal distance of origin L0.start
  measures "d911" horizontal distance of L0.start L0.end
  measures "d912" vertical distance of L0.end L1.end
extrude "Drain slot 11''" cut sketch "草图12 (6)" along normal blind 4 bodies 14 in component "R1_RemovableGrate"
ref_plane "工作平面13" through (0, 0, 36) normal (0, 0, 1) x (1, 0, 0) in component "R1_RemovableGrate"
sketch "草图13 (6)" plane through (0, 0, 36) normal (0, 0, 1) x (1, 0, 0) in component "R1_RemovableGrate"
  line L0 (649, 132.7) -> (665, 132.7)
  line L1 (665, 132.7) -> (665, 137.7)
  line L2 (665, 137.7) -> (649, 137.7)
  line L3 (649, 137.7) -> (649, 132.7)
  dimension "d917" = 649
  dimension "d918" = 132.7
  dimension "d919" = 16
  dimension "d920" = 5
  constraint horizontal L0
  constraint vertical L1
  constraint horizontal L2
  constraint vertical L3
  measures "d917" horizontal distance of origin L0.start
  measures "d918" vertical distance of origin L0.start
  measures "d919" horizontal distance of L0.start L0.end
  measures "d920" vertical distance of L0.end L1.end
extrude "Finger lift notch''" cut sketch "草图13 (6)" along normal blind 4 bodies 14 in component "R1_RemovableGrate"
ref_plane "工作平面1" through (0, 0, 0) normal (0, 0, 1) x (1, 0, 0) in component "R1_Foot_00"
sketch "草图1 (15)" plane through (0, 0, 0) normal (0, 0, 1) x (1, 0, 0) in component "R1_Foot_00"
  line L0 (593, 53) -> (609, 53)
  line L1 (609, 53) -> (609, 69)
  line L2 (609, 69) -> (593, 69)
  line L3 (593, 69) -> (593, 53)
  dimension "d925" = 593
  dimension "d926" = 53
  dimension "d927" = 16
  dimension "d928" = 16
  constraint horizontal L0
  constraint vertical L1
  constraint horizontal L2
  constraint vertical L3
  measures "d925" horizontal distance of origin L0.start
  measures "d926" vertical distance of origin L0.start
  measures "d927" horizontal distance of L0.start L0.end
  measures "d928" vertical distance of L0.end L1.end
extrude "Foot base''''''''" add sketch "草图1 (15)" along normal blind 20 separate body makes body 15 in component "R1_Foot_00"
ref_plane "工作平面2" through (0, 0, 20) normal (0, 0, 1) x (1, 0, 0) in component "R1_Foot_00"
sketch "草图2 (15)" plane through (0, 0, 20) normal (0, 0, 1) x (1, 0, 0) in component "R1_Foot_00"
  line L0 (597, 57) -> (605, 57)
  line L1 (605, 57) -> (605, 65)
  line L2 (605, 65) -> (597, 65)
  line L3 (597, 65) -> (597, 57)
  dimension "d933" = 597
  dimension "d934" = 57
  dimension "d935" = 8
  dimension "d936" = 8
  constraint horizontal L0
  constraint vertical L1
  constraint horizontal L2
  constraint vertical L3
  measures "d933" horizontal distance of origin L0.start
  measures "d934" vertical distance of origin L0.start
  measures "d935" horizontal distance of L0.start L0.end
  measures "d936" vertical distance of L0.end L1.end
extrude "Locating peg''''''''" add sketch "草图2 (15)" along normal blind 1.5 bodies 15 in component "R1_Foot_00"
ref_plane "工作平面1" through (0, 0, 0) normal (0, 0, 1) x (1, 0, 0) in component "R1_Foot_01"
sketch "草图1 (16)" plane through (0, 0, 0) normal (0, 0, 1) x (1, 0, 0) in component "R1_Foot_01"
  line L0 (593, 115) -> (609, 115)
  line L1 (609, 115) -> (609, 131)
  line L2 (609, 131) -> (593, 131)
  line L3 (593, 131) -> (593, 115)
  dimension "d941" = 593
  dimension "d942" = 115
  dimension "d943" = 16
  dimension "d944" = 16
  constraint horizontal L0
  constraint vertical L1
  constraint horizontal L2
  constraint vertical L3
  measures "d941" horizontal distance of origin L0.start
  measures "d942" vertical distance of origin L0.start
  measures "d943" horizontal distance of L0.start L0.end
  measures "d944" vertical distance of L0.end L1.end
extrude "Foot base'''''''''" add sketch "草图1 (16)" along normal blind 20 separate body makes body 16 in component "R1_Foot_01"
ref_plane "工作平面2" through (0, 0, 20) normal (0, 0, 1) x (1, 0, 0) in component "R1_Foot_01"
sketch "草图2 (16)" plane through (0, 0, 20) normal (0, 0, 1) x (1, 0, 0) in component "R1_Foot_01"
  line L0 (597, 119) -> (605, 119)
  line L1 (605, 119) -> (605, 127)
  line L2 (605, 127) -> (597, 127)
  line L3 (597, 127) -> (597, 119)
  dimension "d949" = 597
  dimension "d950" = 119
  dimension "d951" = 8
  dimension "d952" = 8
  constraint horizontal L0
  constraint vertical L1
  constraint horizontal L2
  constraint vertical L3
  measures "d949" horizontal distance of origin L0.start
  measures "d950" vertical distance of origin L0.start
  measures "d951" horizontal distance of L0.start L0.end
  measures "d952" vertical distance of L0.end L1.end
extrude "Locating peg'''''''''" add sketch "草图2 (16)" along normal blind 1.5 bodies 16 in component "R1_Foot_01"
ref_plane "工作平面1" through (0, 0, 0) normal (0, 0, 1) x (1, 0, 0) in component "R1_Foot_10"
sketch "草图1 (17)" plane through (0, 0, 0) normal (0, 0, 1) x (1, 0, 0) in component "R1_Foot_10"
  line L0 (705, 53) -> (721, 53)
  line L1 (721, 53) -> (721, 69)
  line L2 (721, 69) -> (705, 69)
  line L3 (705, 69) -> (705, 53)
  dimension "d957" = 705
  dimension "d958" = 53
  dimension "d959" = 16
  dimension "d960" = 16
  constraint horizontal L0
  constraint vertical L1
  constraint horizontal L2
  constraint vertical L3
  measures "d957" horizontal distance of origin L0.start
  measures "d958" vertical distance of origin L0.start
  measures "d959" horizontal distance of L0.start L0.end
  measures "d960" vertical distance of L0.end L1.end
extrude "Foot base''''''''''" add sketch "草图1 (17)" along normal blind 20 separate body makes body 17 in component "R1_Foot_10"
ref_plane "工作平面2" through (0, 0, 20) normal (0, 0, 1) x (1, 0, 0) in component "R1_Foot_10"
sketch "草图2 (17)" plane through (0, 0, 20) normal (0, 0, 1) x (1, 0, 0) in component "R1_Foot_10"
  line L0 (709, 57) -> (717, 57)
  line L1 (717, 57) -> (717, 65)
  line L2 (717, 65) -> (709, 65)
  line L3 (709, 65) -> (709, 57)
  dimension "d965" = 709
  dimension "d966" = 57
  dimension "d967" = 8
  dimension "d968" = 8
  constraint horizontal L0
  constraint vertical L1
  constraint horizontal L2
  constraint vertical L3
  measures "d965" horizontal distance of origin L0.start
  measures "d966" vertical distance of origin L0.start
  measures "d967" horizontal distance of L0.start L0.end
  measures "d968" vertical distance of L0.end L1.end
extrude "Locating peg''''''''''" add sketch "草图2 (17)" along normal blind 1.5 bodies 17 in component "R1_Foot_10"
ref_plane "工作平面1" through (0, 0, 0) normal (0, 0, 1) x (1, 0, 0) in component "R1_Foot_11"
sketch "草图1 (18)" plane through (0, 0, 0) normal (0, 0, 1) x (1, 0, 0) in component "R1_Foot_11"
  line L0 (705, 115) -> (721, 115)
  line L1 (721, 115) -> (721, 131)
  line L2 (721, 131) -> (705, 131)
  line L3 (705, 131) -> (705, 115)
  dimension "d973" = 705
  dimension "d974" = 115
  dimension "d975" = 16
  dimension "d976" = 16
  constraint horizontal L0
  constraint vertical L1
  constraint horizontal L2
  constraint vertical L3
  measures "d973" horizontal distance of origin L0.start
  measures "d974" vertical distance of origin L0.start
  measures "d975" horizontal distance of L0.start L0.end
  measures "d976" vertical distance of L0.end L1.end
extrude "Foot base'''''''''''" add sketch "草图1 (18)" along normal blind 20 separate body makes body 18 in component "R1_Foot_11"
ref_plane "工作平面2" through (0, 0, 20) normal (0, 0, 1) x (1, 0, 0) in component "R1_Foot_11"
sketch "草图2 (18)" plane through (0, 0, 20) normal (0, 0, 1) x (1, 0, 0) in component "R1_Foot_11"
  line L0 (709, 119) -> (717, 119)
  line L1 (717, 119) -> (717, 127)
  line L2 (717, 127) -> (709, 127)
  line L3 (709, 127) -> (709, 119)
  dimension "d981" = 709
  dimension "d982" = 119
  dimension "d983" = 8
  dimension "d984" = 8
  constraint horizontal L0
  constraint vertical L1
  constraint horizontal L2
  constraint vertical L3
  measures "d981" horizontal distance of origin L0.start
  measures "d982" vertical distance of origin L0.start
  measures "d983" horizontal distance of L0.start L0.end
  measures "d984" vertical distance of L0.end L1.end
extrude "Locating peg'''''''''''" add sketch "草图2 (18)" along normal blind 1.5 bodies 18 in component "R1_Foot_11"
ref_plane "工作平面1" through (0, 0, 20) normal (0, 0, 1) x (1, 0, 0) in component "R2_DrainPan"
sketch "草图1 (19)" plane through (0, 0, 20) normal (0, 0, 1) x (1, 0, 0) in component "R2_DrainPan"
  line L0 (726, 50) -> (860, 50)
  line L1 (860, 50) -> (860, 140)
  line L2 (860, 140) -> (726, 140)
  line L3 (726, 140) -> (726, 50)
  dimension "d989" = 726
  dimension "d990" = 50
  dimension "d991" = 134
  dimension "d992" = 90
  constraint horizontal L0
  constraint vertical L1
  constraint horizontal L2
  constraint vertical L3
  measures "d989" horizontal distance of origin L0.start
  measures "d990" vertical distance of origin L0.start
  measures "d991" horizontal distance of L0.start L0.end
  measures "d992" vertical distance of L0.end L1.end
extrude "Pan blank'''" add sketch "草图1 (19)" along normal blind 20 separate body makes body 19 in component "R2_DrainPan"
fillet "Outside corner rounds'''" radius 3 4 edges at (726, 140, 30) (860, 140, 30) (860, 50, 30) (726, 50, 30) on bodies 19 in component "R2_DrainPan"
ref_plane "工作平面2" through (729, 0, 0) normal (1, 0, 0) x (0, 1, 0) in component "R2_DrainPan"
sketch "草图2 (19)" plane through (729, 0, 0) normal (1, 0, 0) x (0, 0, -1) in component "R2_DrainPan"
  line L0 (-30.8318, 53) -> (-24.958, 137)
  line L1 (-24.958, 137) -> (-41, 137)
  line L2 (-41, 137) -> (-41, 53)
  line L3 (-41, 53) -> (-30.8318, 53)
  dimension "d999" = 30.8318
  dimension "d1001" = 24.958
  dimension "d1003" = 41
  constraint horizontal L1
  constraint vertical L2
  constraint horizontal L3
  measures "d999" horizontal distance of origin L0.start
  measures "d1001" horizontal distance of origin L0.end
  measures "d1003" horizontal distance of origin L1.end
extrude "Sloped catch cavity'''" cut sketch "草图2 (19)" along normal blind 128 bodies 19 in component "R2_DrainPan"
ref_plane "工作平面3" through (727, 0, 0) normal (1, 0, 0) x (0, 1, 0) in component "R2_DrainPan"
sketch "草图3 (7)" plane through (727, 0, 0) normal (1, 0, 0) x (0, 0, -1) in component "R2_DrainPan"
  line L0 (-20, 137) -> (-20, 165)
  line L1 (-20, 165) -> (-23, 165)
  line L2 (-23, 165) -> (-24.958, 137)
  line L3 (-24.958, 137) -> (-20, 137)
  dimension "d1011" = 23
  dimension "d1012" = 24.958
  constraint vertical L0
  constraint horizontal L1
  constraint horizontal L3
  measures "d1011" horizontal distance of origin L1.end
  measures "d1012" horizontal distance of origin L2.end
extrude "Drain tongue floor'''" add sketch "草图3 (7)" along normal blind 34 bodies 19 in component "R2_DrainPan"